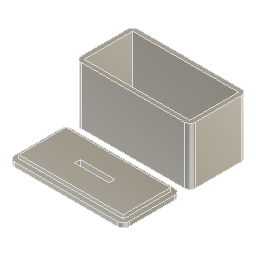
Копилка от ПЭС (Autodesk Fusion 360 design; units mm, degrees)
Autodesk Fusion 360 part; units mm, degrees
sketch "Sketch4" plane through (0, 0, 0) normal (0, 0, 1) x (1, 0, 0)
  line L0 (40, -20) -> (-40, -20)
  line L1 (-40, -20) -> (-40, 20)
  line L2 (-40, 20) -> (40, 20)
  line L3 (40, 20) -> (40, -20)
  line L4 (40, -20) -> (-40, 20) construction
  line L5 (-40, -20) -> (40, 20) construction
  line L6 (37, -17) -> (-37, -17)
  line L7 (-37, -17) -> (-37, 17)
  line L8 (-37, 17) -> (37, 17)
  line L9 (37, 17) -> (37, -17)
  dimension "d8" = 3
  constraint horizontal L0
  constraint perpendicular L0 L1
  constraint parallel L0 L2
  constraint parallel L1 L3
  constraint coincident L4 origin
  constraint coincident L5 origin
extrude "Extrude3" add sketch "Sketch4" along normal blind 3 contours L0 L1 L2 L3 | L6 L7 L8 L9 makes body 1
extrude "Extrude4" add sketch "Sketch4" along normal blind 40 bodies 1
sketch "Sketch5" plane through (0, 0, 0) normal (0, 0, 1) x (1, 0, 0)
  line L0 (40, -20) -> (-40, -20)
  line L1 (-40, -20) -> (-40, 20)
  line L2 (-40, 20) -> (40, 20)
  line L3 (40, 20) -> (40, -20)
  line L4 (40, -20) -> (-40, 20) construction
  line L5 (-40, -20) -> (40, 20) construction
  line L6 (36.5, -16.5) -> (-36.5, -16.5)
  line L7 (-36.5, -16.5) -> (-36.5, 16.5)
  line L8 (-36.5, 16.5) -> (36.5, 16.5)
  line L9 (36.5, 16.5) -> (36.5, -16.5)
  line L10 (12, -2) -> (-12, -2)
  line L11 (-12, -2) -> (-12, 2)
  line L12 (-12, 2) -> (12, 2)
  line L13 (12, 2) -> (12, -2)
  line L14 (12, -2) -> (-12, 2) construction
  line L15 (-12, -2) -> (12, 2) construction
  dimension "d13" = 80
  dimension "d14" = 40
  dimension "d15" = 3.5
  constraint horizontal L0
  constraint perpendicular L0 L1
  constraint parallel L0 L2
  constraint parallel L1 L3
  constraint coincident L4 origin
  constraint coincident L5 origin
  constraint horizontal L10
  constraint perpendicular L10 L11
  constraint parallel L10 L12
  constraint parallel L11 L13
  constraint coincident L14 origin
  constraint coincident L15 origin
  measures "d13" distance of L1.end L2.end
  measures "d14" distance of L0.end L1.end
extrude "Extrude5" add sketch "Sketch5" along normal blind 3 separate body contours L0 L1 L2 L3 | L6 L7 L8 L9 makes body 2
extrude "Extrude6" add sketch "Sketch5" along normal blind 5.5 contours L6 L7 L8 L9 bodies 2
move_body "Move1" bodies 2 to x (1, 0, 0) y (0, -1, 0) z (0, 0, -1) at (0, 0, 51)
fillet "Fillet1" radius 4 8 edges at (-40, -20, 20) (40, -20, 20) (40, 20, 20) (-40, 20, 20) (-40, -20, 49.5) (40, 20, 49.5) (40, -20, 49.5) (-40, 20, 49.5) on bodies 1 2
move_body "Move2" bodies 2 to x (1, 0, 0) y (0, -1, 0) z (0, 0, -1) at (0, -46.5663, 51)
